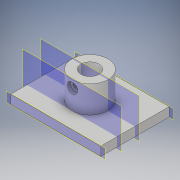
# Autodesk Inventor part: Laserhalter Unterteil 29112018
Saved by Autodesk Inventor 2018.3 (Build 223284000, 284)
## iProperties
Created: 2018-11-22
Part Number: Laserhalter Unterteil 29112018
Material: Generisch
Document SubType Name: Modeling
Designer: pgmadmin
Density: 1 g/cm^3
Appearance: Vorgabe
Author: pgmadmin
Autodesk Inventor part; units mm, degrees
ref_plane "YZ Plane" through (0, 0, 0) normal (1, 0, 0) x (0, 1, 0)
ref_plane "XY Plane" through (0, 0, 0) normal (0, 0, 1) x (1, 0, 0)
sketch "Skizze1" plane through (0, 0, 0) normal (0, 0, 1) x (1, 0, 0)
  line L0 (-25, -19) -> (25, -19)
  line L1 (25, -19) -> (25, 19)
  line L2 (25, 19) -> (-25, 19)
  line L3 (-25, 19) -> (-25, -19)
  line L4 (-25, -19) -> (25, 19) construction
  line L5 (25, -19) -> (-25, 19) construction
  point P0 (0, 0)
  dimension "d0" = 50
  dimension "d1" = 38
  constraints: 12 end point, 2 midpoint, 2 parallel, 1 horizontal, 1 perpendicular
  measures "d0" distance of L1.end L2.end
  measures "d1" distance of L0.end L1.end
extrude "Extrusion1" add sketch "Skizze1" along normal blind 5
sketch "Skizze2" plane through (0, 0, 5) normal (0, 0, 1) x (1, 0, 0)
  point P0 (0, 0)
ref_plane "Arbeitsebene1" through (0, 19, 0) normal (0, 1, 0) x (-1, 0, 0)
ref_plane "Arbeitsebene2" through (0, -19, 0) normal (0, 1, 0) x (-1, 0, 0)
sketch "Skizze4" plane through (0, 0, 5) normal (0, 0, 1) x (1, 0, 0)
  circle A0 centre (0, 0) radius 10
  circle A1 centre (0, 0) radius 5
  dimension "d12" = 20
  dimension "d13" = 10
  constraints: 2 centre point, 2 coincident
  measures "d12" diameter of A0
  measures "d13" diameter of A1
extrude "Extrusion2" add sketch "Skizze4" along normal blind 15
ref_plane "Arbeitsebene3" through (0, -10, 0) normal (0, 1, 0) x (-1, 0, 0)
sketch "Skizze5" plane through (0, -10, 0) normal (0, 1, 0) x (-1, 0, 0)
  line L0 (10, 20) -> (-10, 20) projected
  point P0 (0, 0)
  point P1 (0, 16)
  dimension "d17" = 4
  measures "d17" distance from line of point (0, 16) L0
hole "Bohrung1" at (0, -10, 16) direction (0, 1, 0) diameter 3 depth 8 tip angle 118 counterbore diameter 5.68 counterbore depth 2
sketch "Skizze6" plane through (0, -10, 0) normal (0, 1, 0) x (-1, 0, 0)
  point P0 (0, 0)
sketch "Skizze7" plane through (0, 0, 0) normal (0, 0, -1) x (-1, 0, 0)
  circle A0 centre (0, 0) radius 2.5
  dimension "d25" = 5
  constraints: 2 coincident, 1 centre point
  measures "d25" diameter of A0
hole "Bohrung2" at (0, 0, 0) direction (0, 0, 1) diameter 5 depth 5 tip angle 118
